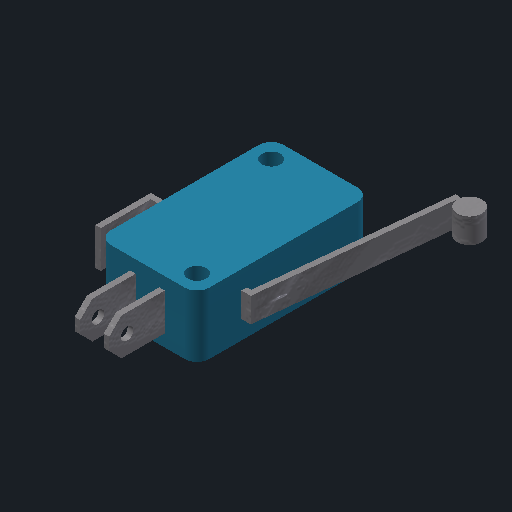
# Autodesk Inventor part: FIN_DE_CARRERA
Saved by Autodesk Inventor 2024.3 (Build 283343000, 343)
## iProperties
Created: 2024-07-19
Part Number: FIN_DE_CARRERA
Material: Steel, Mild, Welded
Document SubType Name: Modeling
Designer: Niler
Density: 7.85 g/cm^3
Appearance: Weld - Steel Mild
Author: Niler
Autodesk Inventor part; units mm, degrees
ref_plane "YZ Plane" through (0, 0, 0) normal (1, 0, 0) x (0, 1, 0)
ref_plane "XZ Plane" through (0, 0, 0) normal (0, 1, 0) x (-1, 0, 0)
ref_plane "XY Plane" through (0, 0, 0) normal (0, 0, 1) x (1, 0, 0)
sketch "Sketch1" plane through (0, 0, 0) normal (0, 1, 0) x (-1, 0, 0)
  line L0 (-8, 14) -> (8, 14)
  line L1 (8, 14) -> (8, -14)
  line L2 (8, -14) -> (-8, -14)
  line L3 (-8, -14) -> (-8, 14)
  line L4 (-8, 14) -> (8, -14) construction
  line L5 (8, 14) -> (-8, -14) construction
  point P0 (0, 0)
  dimension "d0" = 16
  dimension "d1" = 28
  constraints: 12 end point, 2 midpoint, 2 parallel, 1 horizontal, 1 perpendicular
  measures "d0" distance of L1.end L2.end
  measures "d1" distance of L0.end L1.end
extrude "Extrusion1" add sketch "Sketch1" along normal mid plane 10
fillet "Fillet1" radius 2 4 edges at (8, 0, 14) (8, 0, -14) (-8, 0, 14) (-8, 0, -14)
sketch "Sketch2" plane through (0, 5, 0) normal (0, 1, 0) x (1, 0, 0)
  arc A0 (-6, 14) -> (-8, 12) centre (-6, 12) ccw projected
  line L0 (-8, 12) -> (-8, -12) projected
  arc A1 (-8, -12) -> (-6, -14) centre (-6, -12) ccw projected
  line L1 (-6, -14) -> (6, -14) projected
  arc A2 (6, -14) -> (8, -12) centre (6, -12) ccw projected
  line L2 (8, -12) -> (8, 12) projected
  arc A3 (8, 12) -> (6, 14) centre (6, 12) ccw projected
  line L3 (6, 14) -> (-6, 14) projected
  circle A4 centre (-5, 11) radius 1.5
  circle A5 centre (5, -11) radius 1.5
  point P0 (0, 0)
  dimension "d5" = 3
  dimension "d6" = 3
  dimension "d7" = 3
  dimension "d8" = 3
  dimension "d9" = 3
  constraints: 2 centre point, 1 equal radius
  measures "d5" distance from line of L0 A4.centre
  measures "d6" distance from line of L3 A4.centre
  measures "d7" diameter of A4
  measures "d8" distance from line of L1 A5.centre
  measures "d9" distance from line of L2 A5.centre
extrude "Extrusion2" cut sketch "Sketch2" against normal blind 10 contours A4 | A5
sketch "Sketch3" plane through (-6, -5, 14) normal (0, 0, 1) x (1, 0, 0)
  line L0 (0, 0) -> (0, 10) projected
  line L1 (12, 0) -> (0, 0) projected
  line L2 (12, 10) -> (12, 0) projected
  line L3 (0, 10) -> (12, 10) projected
  line L4 (3.2, 10) -> (4.1, 10)
  line L5 (4.1, 10) -> (4.1, 0)
  line L6 (4.1, 0) -> (3.2, 0)
  line L7 (3.2, 0) -> (3.2, 10)
  line L8 (8.8, 10) -> (7.9, 10)
  line L9 (7.9, 10) -> (7.9, 0)
  line L10 (7.9, 0) -> (8.8, 0)
  line L11 (8.8, 0) -> (8.8, 10)
  line L12 (1, 2) -> (11, 2)
  line L13 (11, 2) -> (11, 8) construction
  line L14 (11, 8) -> (1, 8)
  line L15 (1, 8) -> (1, 2) construction
  point P0 (6, 5)
  point P1 (8.8, 8)
  point P2 (7.9, 8)
  point P3 (7.9, 2)
  point P4 (8.8, 2)
  point P5 (4.1, 8)
  point P6 (3.2, 8)
  point P7 (3.2, 2)
  point P8 (4.1, 2)
  point P9 (11, 5)
  point P10 (12, 5)
  dimension "d12" = 0.9
  dimension "d14" = 10
  dimension "d15" = 6
  constraints: 24 end point, 4 parallel, 2 horizontal, 2 midpoint, 2 perpendicular, 2 point on line, 1 horizontal alignment
  measures "d12" distance between parallel lines of L5 L7
  measures "d14" distance of L14.end L13.end
  measures "d15" distance of L13.end L12.end
extrude "Extrusion3" add sketch "Sketch3" along normal blind 9 contours L7 L14 L5 L12 | L9 L14 L11 L12
sketch "Sketch4" plane through (-2.8, -3, 14) normal (-1, 0, 0) x (0, 0, 1)
  line L0 (0, 0) -> (0, 6) projected
  line L1 (9, 6) -> (9, 0) projected
  circle A0 centre (6.0959, 3) radius 1
  line L2 (0, 0) -> (9, 0) projected
  line L3 (0, 6) -> (9, 6) projected
  point P0 (-14, 3)
  point P1 (9, 3)
  dimension "d18" = 2
  constraints: 1 centre point, 1 horizontal alignment, 1 midpoint
  measures "d18" diameter of A0
extrude "Extrusion4" cut sketch "Sketch4" against normal through all contours A0
chamfer "Chamfer1" distance 2 angle 45 4 edges at (-2.35, 3, 23) (2.35, 3, 23) (2.35, -3, 23) (-2.35, -3, 23)
sketch "Sketch5" plane through (0, 0, 0) normal (0, 1, 0) x (-1, 0, 0)
  circle A0 centre (-5, 11) radius 1.5 projected
  circle A1 centre (5, -11) radius 1.5 projected
  arc A2 (6, -14) -> (8, -12) centre (6, -12) ccw projected
  line L0 (8, -12) -> (8, 12) projected
  arc A3 (8, 12) -> (6, 14) centre (6, 12) ccw projected
  line L1 (6, 14) -> (-6, 14) projected
  arc A4 (-6, 14) -> (-8, 12) centre (-6, 12) ccw projected
  line L2 (-8, 12) -> (-8, -12) projected
  arc A5 (-8, -12) -> (-6, -14) centre (-6, -12) ccw projected
  line L3 (-6, -14) -> (6, -14) projected
  line L4 (-8, 6.8206) -> (-9.5, 6.8206)
  line L5 (-9.5, 6.8206) -> (-12.7296, -23.9071)
  line L6 (-11.8345, -24.0012) -> (-8.6896, 5.9206)
  line L7 (-8.6896, 5.9206) -> (-8, 5.9206)
  line L8 (-11.8345, -24.0012) -> (-12.7296, -23.9071)
  line L9 (-12.7296, -23.9071) -> (-14.7187, -23.6981)
  line L10 (-14.7187, -23.6981) -> (-14.6555, -23.0969)
  line L11 (-14.6555, -23.0969) -> (-12.6664, -23.306)
  circle A6 centre (-14.6871, -23.3975) radius 2
  line L12 (-8, 12) -> (-8, -12) projected
  point P0 (0, 0)
  point P1 (-12.6893, -23.3036)
  point P2 (-12.7525, -23.9047)
  dimension "d24" = 0.9
  dimension "d25" = 4
  dimension "d26" = 2
  dimension "d27" = 6
  dimension "d28" = 1.5
  constraints: 16 end point, 4 perpendicular, 4 point on line, 1 centre point, 1 midpoint, 1 other
  measures "d24" distance between parallel lines of L5 L6
  measures "d25" diameter of A6
  measures "d26" distance of L5.end L9.end
  measures "d27" angle of L2 L6
  measures "d28" distance of L4.start L4.end
extrude "Extrusion5" add sketch "Sketch5" along normal mid plane 4 contours L7 L6 L8 L5 L4 L2 | L5 A6 L11 | L9 A6 L5 | A6 L9 L10 L11 | L11 L10 L9 A6
sketch "Sketch6" plane through (0, 0, 0) normal (0, 1, 0) x (-1, 0, 0)
  line L0 (8, -12) -> (8, 12) projected
  line L1 (8, 1.4634) -> (12, 1.4634)
  line L2 (12, 1.4634) -> (12, 2.3634)
  line L3 (12, 2.3634) -> (8, 2.3634)
  line L4 (8, 2.3634) -> (8, 1.4634)
  line L5 (12, 2.3634) -> (11.1, 2.3634)
  line L6 (11.1, 2.3634) -> (11.1, 10.4634)
  line L7 (11.1, 10.4634) -> (12, 10.4634)
  line L8 (12, 10.4634) -> (12, 2.3634)
  point P0 (0, 0)
  dimension "d31" = 4
  dimension "d32" = 0.9
  dimension "d33" = 0.9
  dimension "d34" = 9
  constraints: 16 end point, 4 parallel, 2 horizontal, 2 perpendicular, 1 point on line
  measures "d31" distance of L1.start L1.end
  measures "d32" distance between parallel lines of L1 L3
  measures "d33" distance between parallel lines of L8 L6
  measures "d34" distance between parallel lines of L7 L1
extrude "Extrusion6" add sketch "Sketch6" along normal mid plane 6
body "Solid1"
